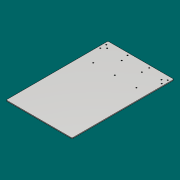
# Autodesk Inventor part: kpd_70_plate
Saved by Autodesk Inventor 2018 (Build 220112000, 112)
## iProperties
Created: 2022-01-26
Part Number: kpd_70_plate
Material: アルミニウム 6061
Document SubType Name: Modeling
Designer: gisen
Density: 2.7 g/cm^3
Appearance: アルミニウム - フラット
Author: gisen
Autodesk Inventor part; units mm, degrees
ref_plane "YZ Plane" through (0, 0, 0) normal (1, 0, 0) x (0, 1, 0)
ref_plane "XZ Plane" through (0, 0, 0) normal (0, 1, 0) x (-1, 0, 0)
ref_plane "XY Plane" through (0, 0, 0) normal (0, 0, 1) x (1, 0, 0)
sketch "スケッチ1" plane through (0, 0, 0) normal (0, 0, 1) x (1, 0, 0)
  line L0 (-120.5, 11.775) -> (120.5, 11.775) construction
  line L1 (120.5, 11.775) -> (120.5, -11.775) construction
  line L2 (120.5, -11.775) -> (-120.5, -11.775) construction
  line L3 (-120.5, -11.775) -> (-120.5, 11.775) construction
  circle A0 centre (-120.5, -11.775) radius 1.6
  circle A1 centre (-120.5, 11.775) radius 1.6
  circle A2 centre (-36.5, -11.775) radius 1.6
  circle A3 centre (42.5, -11.775) radius 1.6
  circle A4 centre (120.5, -11.775) radius 1.6
  line L4 (-129.5, 22.275) -> (-129.5, -20.275) construction
  line L5 (-129.5, 22.275) -> (129.5, 22.275) construction
  line L6 (129.5, 22.275) -> (129.5, -20.275) construction
  line L7 (129.5, -20.275) -> (-129.5, -20.275) construction
  circle A5 centre (-42.5, 17.275) radius 1.6
  circle A6 centre (42.5, 17.275) radius 1.6
  circle A7 centre (120.5, 11.775) radius 1.6
  line L8 (-129.5, -20.275) -> (129.5, -20.275) construction
  line L9 (129.5, -20.275) -> (129.5, 27.275)
  line L10 (129.5, 27.275) -> (-129.5, 27.275)
  line L11 (-129.5, 27.275) -> (-129.5, -20.275)
  line L12 (-129.5, -20.275) -> (-129.5, -372.725)
  line L13 (-129.5, -372.725) -> (129.5, -372.725)
  line L14 (129.5, -372.725) -> (129.5, -20.275)
  line L15 (-129.5, -75.225) -> (129.5, -75.225) construction
  line L16 (0, 27.275) -> (0, -75.225) construction
  circle A8 centre (0, -75.225) radius 2.25
  circle A9 centre (-84.75, -75.225) radius 2.25
  circle A10 centre (84.75, -75.225) radius 2.25
  line L17 (-106.75, 1.275) -> (106.75, 1.275) construction
  circle A11 centre (-106.75, 1.275) radius 2.25
  circle A12 centre (106.75, 1.275) radius 2.25
  point P0 (0, 0)
  point P1 (-120.5, 0)
  point P2 (0, 11.775)
  point P3 (0, 1.275)
  dimension "d0" = 23.55
  dimension "d1" = 84
  dimension "d3" = 79
  dimension "d4" = 78
  dimension "d5" = 3.2
  dimension "d6" = 9
  dimension "d7" = 9
  dimension "d8" = 8.5
  dimension "d9" = 10.5
  dimension "d10" = 5.5
  dimension "d11" = 78.1937
  dimension "d12" = 78.1937
  dimension "d13" = 78
  dimension "d14" = 85
  dimension "d15" = 78
  dimension "d16" = 5
  dimension "d24" = 400
  dimension "d26" = 97.5
  dimension "d27" = 4.5
  dimension "d28" = 169.5
  dimension "d29" = 84.75
  dimension "d30" = 213.5
  dimension "d31" = 21
  constraints: 36 end point, 13 centre point, 11 coincident, 11 equal radius, 7 perpendicular, 6 point on line, 5 midpoint, 4 horizontal, 4 parallel, 2 horizontal alignment, 2 vertical, 2 vertical alignment
  measures "d0" distance of L2.end L0.start
  measures "d1" distance of point (-36.5, -11.775) L2.end
  measures "d3" distance of point (42.5, -11.775) point (-36.5, -11.775)
  measures "d4" distance from line of L1 point (42.5, -11.775)
  measures "d5" diameter of A0
  measures "d6" distance between parallel lines of L3 L4
  measures "d7" distance between parallel lines of L6 L1
  measures "d8" distance between parallel lines of L7 L2
  measures "d9" distance between parallel lines of L0 L5
  measures "d10" distance from line of L0 point (-42.5, 17.275)
  measures "d11" distance of point (-42.5, 17.275) L0.start
  measures "d12" distance of L0.end point (42.5, 17.275)
  measures "d13" horizontal distance of point (-42.5, 17.275) L0.start
  measures "d14" distance of point (42.5, 17.275) point (-42.5, 17.275)
  measures "d15" horizontal distance of L0.end A6.centre
  measures "d16" distance between parallel lines of L5 L10
  measures "d24" distance between parallel lines of L13 L10
  measures "d26" distance between parallel lines of L15 L5
  measures "d27" diameter of A8
  measures "d28" distance of A10.centre A9.centre
  measures "d29" distance of A8.centre A9.centre
  measures "d30" distance of L17.start L17.end
  measures "d31" distance between parallel lines of L17 L5
extrude "押し出し1" add sketch "スケッチ1" along normal blind 3
sketch "スケッチ3" plane through (0, 0, 3) normal (0, 0, 1) x (1, 0, 0)
  circle A0 centre (-106.75, 1.275) radius 2.25 construction
  circle A1 centre (106.75, 1.275) radius 2.25 construction
  circle A2 centre (84.75, -75.225) radius 2.25 construction
  circle A3 centre (0, -75.225) radius 2.25 construction
  circle A4 centre (-84.75, -75.225) radius 2.25 construction
  circle A5 centre (-106.75, 1.275) radius 4.25
  circle A6 centre (106.75, 1.275) radius 4.25
  circle A7 centre (84.75, -75.225) radius 4.25
  circle A8 centre (0, -75.225) radius 4.25
  circle A9 centre (-84.75, -75.225) radius 4.25
  point P0 (0, 0)
  dimension "d33" = 8.5
  constraints: 5 centre point, 5 coincident, 4 equal radius
  measures "d33" diameter of A5
extrude "押し出し3" cut sketch "スケッチ3" along normal blind 1.5 from surface at -3
sketch "スケッチ5" plane through (0, 0, 0) normal (0, 0, -1) x (-1, 0, 0)
  circle A0 centre (0, -75.225) radius 4.25 construction
  circle A1 centre (-106.75, 1.275) radius 4.25 construction
  circle A2 centre (106.75, 1.275) radius 4.25 construction
  circle A3 centre (-84.75, -75.225) radius 4.25 construction
  circle A4 centre (84.75, -75.225) radius 4.25 construction
  circle A5 centre (-120.5, 11.775) radius 1.6 construction
  circle A6 centre (-42.5, 17.275) radius 1.6 construction
  circle A7 centre (42.5, 17.275) radius 1.6 construction
  circle A8 centre (-120.5, -11.775) radius 1.6 construction
  circle A9 centre (-42.5, -11.775) radius 1.6 construction
  circle A10 centre (36.5, -11.775) radius 1.6 construction
  circle A11 centre (120.5, 11.775) radius 1.6 construction
  circle A12 centre (120.5, -11.775) radius 1.6 construction
  line L0 (129.5, -372.725) -> (129.5, 27.275) construction
  line L1 (129.5, 27.275) -> (-129.5, 27.275) construction
  line L2 (-129.5, 27.275) -> (-129.5, -372.725) construction
  line L3 (-129.5, -372.725) -> (129.5, -372.725) construction
  circle A13 centre (-120.5, 11.775) radius 2.25
  circle A14 centre (-120.5, -11.775) radius 2.25
  circle A15 centre (-42.5, 17.275) radius 2.25
  circle A16 centre (-42.5, -11.775) radius 2.25
  circle A17 centre (42.5, 17.275) radius 2.25
  circle A18 centre (36.5, -11.775) radius 2.25
  circle A19 centre (120.5, 11.775) radius 2.25
  circle A20 centre (120.5, -11.775) radius 2.25
  circle A21 centre (106.75, 1.275) radius 2.25 projected
  point P0 (0, 0)
  constraints: 8 centre point, 8 coincident, 8 equal radius
extrude "押し出し4" cut sketch "スケッチ5" against normal through all contours A13 | A14 | A15 | A16 | A17 | A18 | A19 | A20
sketch "スケッチ6" plane through (0, 0, 0) normal (0, 0, -1) x (-1, 0, 0)
  circle A0 centre (120.5, 11.775) radius 2.25 construction
  circle A1 centre (42.5, 17.275) radius 2.25 construction
  circle A2 centre (-42.5, 17.275) radius 2.25 construction
  circle A3 centre (-120.5, 11.775) radius 2.25 construction
  circle A4 centre (-120.5, -11.775) radius 2.25 construction
  circle A5 centre (-42.5, -11.775) radius 2.25 construction
  circle A6 centre (36.5, -11.775) radius 2.25 construction
  circle A7 centre (120.5, -11.775) radius 2.25 construction
  circle A8 centre (0, -75.225) radius 4.25 construction
  circle A9 centre (-106.75, 1.275) radius 4.25 construction
  circle A10 centre (106.75, 1.275) radius 4.25 construction
  circle A11 centre (-84.75, -75.225) radius 4.25 construction
  circle A12 centre (84.75, -75.225) radius 4.25 construction
  line L0 (129.5, -372.725) -> (129.5, 27.275) construction
  line L1 (129.5, 27.275) -> (-129.5, 27.275) construction
  line L2 (-129.5, 27.275) -> (-129.5, -372.725) construction
  line L3 (-129.5, -372.725) -> (129.5, -372.725) construction
  circle A13 centre (-120.5, 11.775) radius 4.25
  circle A14 centre (-120.5, -11.775) radius 4.25
  circle A15 centre (-42.5, 17.275) radius 4.25
  circle A16 centre (-42.5, -11.775) radius 4.25
  circle A17 centre (36.5, -11.775) radius 4.25
  circle A18 centre (42.5, 17.275) radius 4.25
  circle A19 centre (120.5, -11.775) radius 4.25
  circle A20 centre (120.5, 11.775) radius 4.25
  circle A21 centre (106.75, 1.275) radius 4.25 projected
  point P0 (0, 0)
  constraints: 8 centre point, 8 coincident, 8 equal radius
extrude "押し出し5" cut sketch "スケッチ6" against normal blind 1.5 contours A13 | A14 | A15 | A16 | A17 | A18 | A19 | A20
fillet "フィレット4" radius 4 4 edges at (129.5, -372.725, 1.5) (-129.5, -372.725, 1.5) (-129.5, 27.275, 1.5) (129.5, 27.275, 1.5)
equation "\"d12\" = d11"
equation "\"d29\" = 0.5 * d28"
